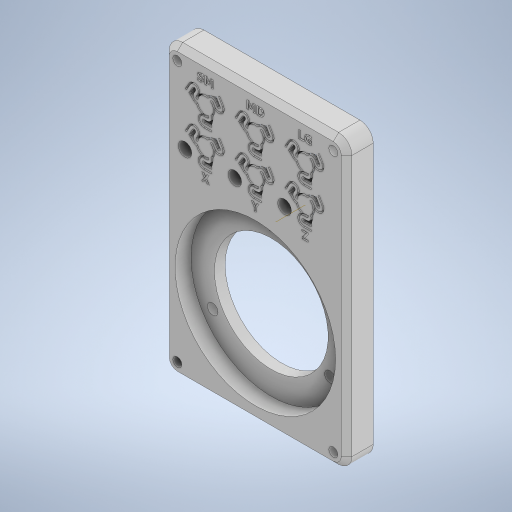
# Autodesk Inventor part: Case Front
Saved by Autodesk Inventor 2023.1 (Build 271208000, 208)
## iProperties
Created: 2022-10-09
Part Number: Case Front
Material: Generic
Document SubType Name: Modeling
Designer: Nick
Density: 1 g/cm^3
Appearance: Default
Author: Nick
Autodesk Inventor part; units mm, degrees
(part 1 of 3)
ref_plane "YZ Plane" through (0, 0, 0) normal (1, 0, 0) x (0, 1, 0)
ref_plane "XZ Plane" through (0, 0, 0) normal (0, 1, 0) x (-1, 0, 0)
ref_plane "XY Plane" through (0, 0, 0) normal (0, 0, 1) x (1, 0, 0)
sketch "Sketch1" plane through (0, 0, 0) normal (0, 0, 1) x (1, 0, 0)
  line L0 (0, 0) -> (68.58, 0)
  line L1 (68.58, 0) -> (68.58, 107.95)
  line L2 (68.58, 107.95) -> (0, 107.95)
  line L3 (0, 107.95) -> (0, 0)
  dimension "d0" = 68.58
  dimension "d1" = 107.95
  constraints: 8 end point, 2 parallel, 1 horizontal, 1 perpendicular
  measures "d0" distance of L2.end L1.end
  measures "d1" distance of L1.end L0.end
extrude "Extrusion1" add sketch "Sketch1" along normal blind 10
sketch "Sketch2" plane through (0, 0, 10) normal (0, 0, 1) x (1, 0, 0)
  circle A0 centre (34.29, 35.56) radius 30.149
  line L0 (0, 0) -> (68.58, 0) projected
  point P0 (34.29, 0)
  dimension "d4" = 60.298
  dimension "d5" = 35.56
  constraints: 1 centre point, 1 midpoint, 1 vertical alignment
  measures "d4" diameter of A0
  measures "d5" distance from line of L0 A0.centre
extrude "Extrusion2" cut sketch "Sketch2" against normal blind 16.9875
sketch "Sketch3" plane through (0, 0, 0) normal (0, 0, -1) x (-1, 0, 0)
  circle A0 centre (-34.29, 35.56) radius 30.149 projected
  circle A1 centre (-34.29, 35.56) radius 21.3606
  point P0 (0, 0)
  dimension "d8" = 42.7212
  constraints: 1 centre point, 1 coincident
  measures "d8" diameter of A1
extrude "Extrusion3" add sketch "Sketch3" against normal blind 4
sketch "Sketch4" plane through (0, 0, 10) normal (0, 0, 1) x (1, 0, 0)
  circle A0 centre (15.59, 80.0195) radius 3
  circle A1 centre (34.29, 80.0195) radius 3
  circle A2 centre (52.99, 93.6395) radius 3
  circle A3 centre (34.29, 93.6395) radius 3
  circle A4 centre (15.59, 93.6395) radius 3
  line L0 (12.59, 96.6395) -> (18.59, 96.6395) construction
  line L1 (18.59, 96.6395) -> (18.59, 90.6395) construction
  line L2 (18.59, 90.6395) -> (12.59, 90.6395) construction
  line L3 (12.59, 90.6395) -> (12.59, 96.6395) construction
  line L4 (31.29, 96.6395) -> (37.29, 96.6395) construction
  line L5 (37.29, 96.6395) -> (37.29, 90.6395) construction
  line L6 (37.29, 90.6395) -> (31.29, 90.6395) construction
  line L7 (31.29, 90.6395) -> (31.29, 96.6395) construction
  line L8 (49.99, 96.6395) -> (55.99, 96.6395) construction
  line L9 (55.99, 96.6395) -> (55.99, 90.6395) construction
  line L10 (55.99, 90.6395) -> (49.99, 90.6395) construction
  line L11 (49.99, 90.6395) -> (49.99, 96.6395) construction
  line L12 (31.29, 83.0195) -> (37.29, 83.0195) construction
  line L13 (37.29, 83.0195) -> (37.29, 77.0195) construction
  line L14 (37.29, 77.0195) -> (31.29, 77.0195) construction
  line L15 (31.29, 77.0195) -> (31.29, 83.0195) construction
  line L16 (12.59, 83.0195) -> (18.59, 83.0195) construction
  line L17 (18.59, 83.0195) -> (18.59, 77.0195) construction
  line L18 (18.59, 77.0195) -> (12.59, 77.0195) construction
  line L19 (12.59, 77.0195) -> (12.59, 83.0195) construction
  line L20 (68.58, 107.95) -> (0, 107.95) construction
  line L21 (17.8543, 65.709) -> (37.2658, 65.709) construction
  circle A5 centre (34.29, 35.56) radius 30.149 construction
  line L22 (27.9805, 81.0411) -> (29.433, 83.5569)
  line L23 (30.7639, 81.3221) -> (31.3989, 82.4219)
  line L24 (27.1145, 81.5411) -> (28.567, 84.0569)
  line L25 (29.8978, 81.8221) -> (30.5328, 82.9219)
  arc A6 (31.3989, 82.4219) -> (28.567, 84.0569) centre (29.9829, 83.2394) ccw
  arc A7 (30.5328, 82.9219) -> (29.433, 83.5569) centre (29.9829, 83.2394) ccw
  arc A8 (29.8978, 81.8221) -> (31.3611, 79.3703) centre (31.3138, 81.0046) ccw
  arc A9 (30.7639, 81.3221) -> (31.3105, 80.3696) centre (31.3138, 81.0046) ccw
  line L26 (34.29, 80.0195) -> (31.0814, 81.872) construction
  line L27 (34.29, 83.0195) -> (34.29, 80.0195) construction
  line L28 (27.1145, 81.5411) -> (27.9805, 81.0411)
  line L29 (26.6814, 81.7911) -> (28.4135, 80.7911)
  line L30 (28.4135, 80.7911) -> (29.866, 83.3069)
  line L31 (30.0998, 83.1719) -> (29.4648, 82.0721)
  arc A10 (30.0998, 83.1719) -> (29.866, 83.3069) centre (29.9829, 83.2394) ccw
  arc A11 (29.4648, 82.0721) -> (31.5152, 78.8791) centre (31.3138, 81.0046) ccw
  arc A12 (31.8319, 82.1719) -> (28.1339, 84.3069) centre (29.9829, 83.2394) ccw
  arc A13 (31.1969, 81.0721) -> (31.442, 80.9622) centre (31.3138, 81.0046) ccw
  line L32 (31.1969, 81.0721) -> (31.8319, 82.1719)
  line L33 (28.1339, 84.3069) -> (26.6814, 81.7911)
  circle A14 centre (52.99, 80.0195) radius 3
  line L34 (49.99, 83.0195) -> (55.99, 83.0195) construction
  line L35 (55.99, 83.0195) -> (55.99, 77.0195) construction
  line L36 (55.99, 77.0195) -> (49.99, 77.0195) construction
  line L37 (49.99, 77.0195) -> (49.99, 83.0195) construction
  line L38 (46.6805, 81.0411) -> (48.133, 83.5569)
  line L39 (49.4639, 81.3221) -> (50.0989, 82.4219)
  line L40 (45.8145, 81.5411) -> (47.267, 84.0569)
  line L41 (48.5978, 81.8221) -> (49.2328, 82.9219)
  arc A15 (50.0989, 82.4219) -> (47.267, 84.0569) centre (48.6829, 83.2394) ccw
  arc A16 (49.2328, 82.9219) -> (48.133, 83.5569) centre (48.6829, 83.2394) ccw
  arc A17 (48.5978, 81.8221) -> (50.0611, 79.3703) centre (50.0138, 81.0046) ccw
  arc A18 (49.4639, 81.3221) -> (50.0105, 80.3696) centre (50.0138, 81.0046) ccw
  line L42 (52.99, 80.0195) -> (49.7814, 81.872) construction
  line L43 (52.99, 83.0195) -> (52.99, 80.0195) construction
  line L44 (45.8145, 81.5411) -> (46.6805, 81.0411)
  line L45 (45.3814, 81.7911) -> (47.1135, 80.7911)
  line L46 (47.1135, 80.7911) -> (48.566, 83.3069)
  line L47 (48.7998, 83.1719) -> (48.1648, 82.0721)
  arc A19 (48.7998, 83.1719) -> (48.566, 83.3069) centre (48.6829, 83.2394) ccw
  arc A20 (48.1648, 82.0721) -> (50.2152, 78.8791) centre (50.0138, 81.0046) ccw
  arc A21 (50.5319, 82.1719) -> (46.8339, 84.3069) centre (48.6829, 83.2394) ccw
  arc A22 (49.8969, 81.0721) -> (50.142, 80.9622) centre (50.0138, 81.0046) ccw
  line L48 (49.8969, 81.0721) -> (50.5319, 82.1719)
  line L49 (46.8339, 84.3069) -> (45.3814, 81.7911)
  circle A23 centre (52.99, 80.0195) radius 3.508
  line L50 (47.1135, 80.7911) -> (48.557, 79.4438)
  point P0 (0, 0)
  point P1 (37.29, 80.0195)
  point P2 (18.59, 80.0195)
  point P3 (18.59, 93.6395)
  point P4 (31.29, 93.6395)
  point P5 (55.99, 93.6395)
  point P6 (34.29, 96.6395)
  point P7 (52.99, 96.6395)
  point P8 (15.59, 96.6395)
  point P9 (15.59, 83.0195)
  point P10 (34.29, 107.95)
  point P11 (27.5475, 81.2911)
  point P12 (55.99, 80.0195)
  point P13 (46.2475, 81.2911)
  point P14 (49.6661, 78.8981)
  point P15 (50.7545, 82.7229)
  point P16 (46.0107, 79.4247)
  dimension "d11" = 7.62
  dimension "d12" = 6
  dimension "d13" = 6
  dimension "d14" = 12.7
  dimension "d15" = 12.7
  dimension "d16" = 11.3105
  dimension "d17" = 11.3105
  dimension "d18" = 1
  dimension "d19" = 60
  dimension "d23" = 1.27
  dimension "d24" = 0.635
  dimension "d25" = 0.5
  dimension "d34" = 6
  dimension "d35" = 6
  dimension "d36" = 1
  dimension "d37" = 60
  dimension "d38" = 1.27
  dimension "d39" = 0.635
  dimension "d40" = 0.5
  dimension "d58" = 0.508
  constraints: 100 end point, 41 point on circle, 30 tangent, 26 parallel, 23 centre point, 19 midpoint, 12 concentric, 10 equal length, 10 perpendicular, 7 collinear, 7 horizontal, 7 vertical alignment, 6 equal radius, 6 horizontal alignment, 2 point on line, 2 vertical
  measures "d11" distance between parallel lines of L12 L6
  measures "d12" distance of L12.start L12.end
  measures "d13" diameter of A1
  measures "d14" distance between parallel lines of L11 L5
  measures "d15" distance between parallel lines of L1 L7
  measures "d16" distance between parallel lines of L20 L4
  measures "d17" distance between parallel lines of L21 L14
  measures "d18" distance between parallel lines of L23 L25
  measures "d19" angle of L27 L26
  measures "d23" distance of L25.start L25.end
  measures "d24" radius of A9
  measures "d25" distance between parallel lines of L30 L22
  measures "d34" distance of L37.end L35.start
  measures "d35" diameter of A14
  measures "d36" distance between parallel lines of L39 L41
  measures "d37" angle of L43 L42
  measures "d38" distance of L41.start L41.end
  measures "d39" radius of A18
  measures "d40" distance between parallel lines of L46 L38
  measures "d58" radial gap between concentric circles of A14 A23
extrude "Extrusion5" cut sketch "Sketch4" against normal through all contours A14 A18 A23 A21 L48 A22 | A20 A23 A17 A14 | A20 L47 A19 L46 L45 L38 A16 L41 A17 A23 | A18 L39 A15 L40 L45 L49 A21 A23 | L50 L46 A19 L47 A20
pattern_circular "Circular Pattern2" count 3 over 360 about axis through (52.99, 80.0195, 10) along (0, 0, 1) of "Extrusion5"
sketch "Sketch6" plane through (0, 0, 10) normal (0, 0, 1) x (1, 0, 0)
  arc A0 (53.8922, 82.8806) -> (53.3898, 82.9927) centre (52.99, 80.0195) ccw projected
  arc A1 (54.7079, 84.1464) -> (53.3898, 82.9927) centre (55.3312, 82.1044) ccw projected
  line L0 (56.5965, 84.7229) -> (57.0295, 84.9729) projected
  line L1 (57.0295, 84.9729) -> (58.482, 82.4571) projected
  arc A2 (57.3822, 81.8221) -> (58.482, 82.4571) centre (57.9321, 82.1396) ccw projected
  line L2 (57.3822, 81.8221) -> (56.7472, 82.9219) projected
  arc A3 (56.7472, 82.9219) -> (53.8922, 82.8806) centre (55.3312, 82.1044) ccw projected
  arc A4 (55.2304, 82.0147) -> (54.7829, 82.4248) centre (52.99, 80.0195) ccw projected
  arc A5 (55.8811, 82.4219) -> (54.7829, 82.4248) centre (55.3312, 82.1044) ccw projected
  line L3 (55.8811, 82.4219) -> (56.5161, 81.3221) projected
  arc A6 (56.5161, 81.3221) -> (59.348, 82.9571) centre (57.9321, 82.1396) ccw projected
  line L4 (59.348, 82.9571) -> (57.8955, 85.4729) projected
  line L5 (57.8955, 85.4729) -> (58.3286, 85.7229) projected
  line L6 (58.3286, 85.7229) -> (59.7811, 83.2071) projected
  arc A7 (56.0831, 81.0721) -> (59.7811, 83.2071) centre (57.9321, 82.1396) ccw projected
  line L7 (56.0831, 81.0721) -> (55.4481, 82.1719) projected
  arc A8 (55.4481, 82.1719) -> (55.2304, 82.0147) centre (55.3312, 82.1044) ccw projected
  arc A9 (55.0167, 77.8076) -> (55.365, 78.1867) centre (52.99, 80.0195) ccw projected
  arc A10 (55.7051, 76.4683) -> (55.365, 78.1867) centre (53.625, 76.9495) ccw projected
  line L8 (55.26, 74.5445) -> (55.26, 74.0445) projected
  line L9 (55.26, 74.0445) -> (52.355, 74.0445) projected
  arc A11 (52.355, 75.3145) -> (52.355, 74.0445) centre (52.355, 74.6795) ccw projected
  line L10 (52.355, 75.3145) -> (53.625, 75.3145) projected
  arc A12 (53.625, 75.3145) -> (55.0167, 77.8076) centre (53.625, 76.9495) ccw projected
  arc A13 (53.5977, 77.0817) -> (54.1766, 77.2641) centre (52.99, 80.0195) ccw projected
  arc A14 (53.625, 76.3145) -> (54.1766, 77.2641) centre (53.625, 76.9495) ccw projected
  line L11 (53.625, 76.3145) -> (52.355, 76.3145) projected
  arc A15 (52.355, 76.3145) -> (52.355, 73.0445) centre (52.355, 74.6795) ccw projected
  line L12 (52.355, 73.0445) -> (55.26, 73.0445) projected
  line L13 (55.26, 73.0445) -> (55.26, 72.5445) projected
  line L14 (55.26, 72.5445) -> (52.355, 72.5445) projected
  arc A16 (52.355, 76.8145) -> (52.355, 72.5445) centre (52.355, 74.6795) ccw projected
  line L15 (52.355, 76.8145) -> (53.625, 76.8145) projected
  arc A17 (53.625, 76.8145) -> (53.5977, 77.0817) centre (53.625, 76.9495) ccw projected
  line L16 (47.1135, 80.7911) -> (46.6805, 81.0411) projected
  line L17 (46.6805, 81.0411) -> (48.133, 83.5569) projected
  arc A18 (49.2328, 82.9219) -> (48.133, 83.5569) centre (48.6829, 83.2394) ccw projected
  line L18 (49.2328, 82.9219) -> (48.5978, 81.8221) projected
  arc A19 (48.5978, 81.8221) -> (50.0611, 79.3703) centre (50.0138, 81.0046) ccw projected
  arc A20 (50.0611, 79.3703) -> (50.2152, 78.8791) centre (52.99, 80.0195) ccw projected
  arc A21 (48.557, 79.4438) -> (50.2152, 78.8791) centre (50.0138, 81.0046) ccw projected
  line L19 (47.267, 84.0569) -> (45.8145, 81.5411) projected
  line L20 (45.8145, 81.5411) -> (45.3814, 81.7911) projected
  line L21 (45.3814, 81.7911) -> (46.8339, 84.3069) projected
  arc A22 (50.5319, 82.1719) -> (46.8339, 84.3069) centre (48.6829, 83.2394) ccw projected
  line L22 (50.5319, 82.1719) -> (49.8969, 81.0721) projected
  arc A23 (49.8969, 81.0721) -> (50.142, 80.9622) centre (50.0138, 81.0046) ccw projected
  arc A24 (50.142, 80.9622) -> (50.0105, 80.3696) centre (52.99, 80.0195) ccw projected
  arc A25 (49.4639, 81.3221) -> (50.0105, 80.3696) centre (50.0138, 81.0046) ccw projected
  line L23 (49.4639, 81.3221) -> (50.0989, 82.4219) projected
  arc A26 (50.0989, 82.4219) -> (47.267, 84.0569) centre (48.6829, 83.2394) ccw projected
  circle A27 centre (34.29, 35.56) radius 30.149 projected
  line L24 (68.58, 0) -> (68.58, 107.95) projected
  line L25 (68.58, 107.95) -> (0, 107.95) projected
  line L26 (0, 107.95) -> (0, 0) projected
  line L27 (0, 0) -> (68.58, 0) projected
  circle A28 centre (52.99, 80.0195) radius 3
  circle A29 centre (52.99, 80.0195) radius 3.508
  line L28 (54.7079, 84.1464) -> (56.5965, 84.7229) projected
  line L29 (55.7051, 76.4683) -> (55.26, 74.5445) projected
  line L30 (48.557, 79.4438) -> (47.1135, 80.7911) projected
  point P0 (53.5977, 77.0817)
  point P1 (50.2152, 78.8791)
  point P2 (49.6661, 78.8981)
  point P3 (51.7665, 76.7318)
  point P4 (55.2304, 82.0147)
  point P5 (55.365, 78.1867)
  point P6 (55.6231, 77.7016)
  point P7 (56.449, 80.6038)
  point P8 (50.142, 80.9622)
  point P9 (53.3898, 82.9927)
  point P10 (53.6808, 83.4588)
  point P11 (50.7545, 82.7229)
  dimension "d59" = 6
  dimension "d60" = 0.508
  constraints: 2 centre point, 1 coincident
  measures "d59" diameter of A28
  measures "d60" radial gap between concentric circles of A28 A29
extrude "Extrusion7" cut sketch "Sketch6" against normal through all contours A28 A23 L22 A22 A29 A1 | A8 L7 A7 A29 A10 A28 | A28 A17 L15 A16 A29 A21
pattern_linear "Rectangular Pattern2" count 3 spacing 18.7 along (-1, 0, 0) count 2 spacing 13.62 along (0, 1, 0) of "Extrusion5", "Circular Pattern2", "Extrusion7"
sketch "Sketch5" plane through (0, 0, 0) normal (0, 0, -1) x (-1, 0, 0)
  line L0 (-66.58, 105.95) -> (-2, 105.95)
  line L1 (-2, 105.95) -> (-2, 65.9374)
  line L2 (-2, 65.9374) -> (-66.58, 65.9374)
  line L3 (-66.58, 65.9374) -> (-66.58, 105.95)
  line L4 (-68.58, 107.95) -> (0, 107.95) projected
  line L5 (0, 107.95) -> (0, 0) projected
  line L6 (-68.58, 0) -> (-68.58, 107.95) projected
  line L7 (-14.955, 72.5445) -> (-17.86, 72.5445) projected
  point P0 (-20.9286, 99.3429)
  dimension "d52" = 2
  dimension "d53" = 2
  dimension "d54" = 2
  dimension "d74" = 6.6071
  dimension "d75" = 6.6071
  constraints: 8 end point, 2 parallel, 1 horizontal, 1 perpendicular
  measures "d52" distance between parallel lines of L4 L0
  measures "d53" distance between parallel lines of L5 L1
  measures "d54" distance between parallel lines of L6 L3
  measures "d74" distance from line of L0 point (-20.929, 99.343)
  measures "d75" distance between parallel lines of L2 L7
extrude "Extrusion6" cut sketch "Sketch5" against normal blind 9
sketch "Sketch7" plane through (0, 0, 10) normal (0, 0, 1) x (1, 0, 0)
  line L0 (11.8335, 71.5445) -> (19.3465, 71.5445) construction
  line L1 (19.3465, 71.5445) -> (19.3465, 68.4965) construction
  line L2 (19.3465, 68.4965) -> (11.8335, 68.4965) construction
  line L3 (11.8335, 68.4965) -> (11.8335, 71.5445) construction
  line L4 (30.5175, 71.5445) -> (38.0625, 71.5445) construction
  line L5 (38.0625, 71.5445) -> (38.0625, 68.4965) construction
  line L6 (38.0625, 68.4965) -> (30.5175, 68.4965) construction
  line L7 (30.5175, 68.4965) -> (30.5175, 71.5445) construction
  line L8 (54.358, 71.5445) -> (51.622, 71.5445) construction
  line L9 (51.622, 71.5445) -> (51.622, 68.4965) construction
  line L10 (51.622, 68.4965) -> (54.358, 68.4965) construction
  line L11 (54.358, 68.4965) -> (54.358, 71.5445) construction
  line L12 (12.8075, 103.4996) -> (18.3725, 103.4996) construction
  line L13 (18.3725, 103.4996) -> (18.3725, 100.3429) construction
  line L14 (18.3725, 100.3429) -> (12.8075, 100.3429) construction
  line L15 (12.8075, 100.3429) -> (12.8075, 103.4996) construction
  line L16 (31.2531, 103.3909) -> (37.3269, 103.3909) construction
  line L17 (37.3269, 103.3909) -> (37.3269, 100.3429) construction
  line L18 (37.3269, 100.3429) -> (31.2531, 100.3429) construction
  line L19 (31.2531, 100.3429) -> (31.2531, 103.3909) construction
  line L20 (50.5484, 103.5045) -> (55.4316, 103.5045) construction
  line L21 (55.4316, 103.5045) -> (55.4316, 100.3429) construction
  line L22 (55.4316, 100.3429) -> (50.5484, 100.3429) construction
  line L23 (50.5484, 100.3429) -> (50.5484, 103.5045) construction
  line L24 (68.58, 0) -> (68.58, 107.95) projected
  line L25 (68.58, 107.95) -> (0, 107.95) projected
  line L26 (0, 107.95) -> (0, 0) projected
  line L27 (0, 0) -> (68.58, 0) projected
  circle A0 centre (34.29, 35.56) radius 30.149 projected
  arc A1 (53.6808, 83.4588) -> (50.7545, 82.7229) centre (52.99, 80.0195) ccw projected
  arc A2 (54.7079, 84.1464) -> (53.6808, 83.4588) centre (55.3312, 82.1044) ccw projected
  line L28 (56.5965, 84.7229) -> (57.0295, 84.9729) projected
  line L29 (57.0295, 84.9729) -> (58.482, 82.4571) projected
  arc A3 (57.3822, 81.8221) -> (58.482, 82.4571) centre (57.9321, 82.1396) ccw projected
  line L30 (57.3822, 81.8221) -> (56.7472, 82.9219) projected
  arc A4 (56.7472, 82.9219) -> (53.8922, 82.8806) centre (55.3312, 82.1044) ccw projected
  arc A5 (53.8922, 82.8806) -> (50.0105, 80.3696) centre (52.99, 80.0195) ccw projected
  arc A6 (49.4639, 81.3221) -> (50.0105, 80.3696) centre (50.0138, 81.0046) ccw projected
  line L31 (49.4639, 81.3221) -> (50.0989, 82.4219) projected
  arc A7 (50.0989, 82.4219) -> (47.267, 84.0569) centre (48.6829, 83.2394) ccw projected
  line L32 (47.267, 84.0569) -> (45.8145, 81.5411) projected
  line L33 (45.8145, 81.5411) -> (45.3814, 81.7911) projected
  line L34 (45.3814, 81.7911) -> (46.8339, 84.3069) projected
  arc A8 (50.7545, 82.7229) -> (46.8339, 84.3069) centre (48.6829, 83.2394) ccw projected
  arc A9 (55.6231, 77.7016) -> (56.449, 80.6038) centre (52.99, 80.0195) ccw projected
  arc A10 (55.7051, 76.4683) -> (55.6231, 77.7016) centre (53.625, 76.9495) ccw projected
  line L35 (55.26, 74.5445) -> (55.26, 74.0445) projected
  line L36 (55.26, 74.0445) -> (52.355, 74.0445) projected
  arc A11 (52.355, 75.3145) -> (52.355, 74.0445) centre (52.355, 74.6795) ccw projected
  line L37 (52.355, 75.3145) -> (53.625, 75.3145) projected
  arc A12 (53.625, 75.3145) -> (55.0167, 77.8076) centre (53.625, 76.9495) ccw projected
  arc A13 (55.0167, 77.8076) -> (54.7829, 82.4248) centre (52.99, 80.0195) ccw projected
  arc A14 (55.8811, 82.4219) -> (54.7829, 82.4248) centre (55.3312, 82.1044) ccw projected
  line L38 (55.8811, 82.4219) -> (56.5161, 81.3221) projected
  arc A15 (56.5161, 81.3221) -> (59.348, 82.9571) centre (57.9321, 82.1396) ccw projected
  line L39 (59.348, 82.9571) -> (57.8955, 85.4729) projected
  line L40 (57.8955, 85.4729) -> (58.3286, 85.7229) projected
  line L41 (58.3286, 85.7229) -> (59.7811, 83.2071) projected
  arc A16 (56.449, 80.6038) -> (59.7811, 83.2071) centre (57.9321, 82.1396) ccw projected
  arc A17 (49.6661, 78.8981) -> (51.7665, 76.7318) centre (52.99, 80.0195) ccw projected
  arc A18 (48.557, 79.4438) -> (49.6661, 78.8981) centre (50.0138, 81.0046) ccw projected
  line L42 (47.1135, 80.7911) -> (46.6805, 81.0411) projected
  line L43 (46.6805, 81.0411) -> (48.133, 83.5569) projected
  arc A19 (49.2328, 82.9219) -> (48.133, 83.5569) centre (48.6829, 83.2394) ccw projected
  line L44 (49.2328, 82.9219) -> (48.5978, 81.8221) projected
  arc A20 (48.5978, 81.8221) -> (50.0611, 79.3703) centre (50.0138, 81.0046) ccw projected
  arc A21 (50.0611, 79.3703) -> (54.1766, 77.2641) centre (52.99, 80.0195) ccw projected
  arc A22 (53.625, 76.3145) -> (54.1766, 77.2641) centre (53.625, 76.9495) ccw projected
  line L45 (53.625, 76.3145) -> (52.355, 76.3145) projected
  arc A23 (52.355, 76.3145) -> (52.355, 73.0445) centre (52.355, 74.6795) ccw projected
  line L46 (52.355, 73.0445) -> (55.26, 73.0445) projected
  line L47 (55.26, 73.0445) -> (55.26, 72.5445) projected
  line L48 (55.26, 72.5445) -> (52.355, 72.5445) projected
  arc A24 (51.7665, 76.7318) -> (52.355, 72.5445) centre (52.355, 74.6795) ccw projected
  arc A25 (31.3611, 79.3703) -> (35.4766, 77.2641) centre (34.29, 80.0195) ccw projected
  arc A26 (34.925, 76.3145) -> (35.4766, 77.2641) centre (34.925, 76.9495) ccw projected
  line L49 (34.925, 76.3145) -> (33.655, 76.3145) projected
  arc A27 (33.655, 76.3145) -> (33.655, 73.0445) centre (33.655, 74.6795) ccw projected
  line L50 (33.655, 73.0445) -> (36.56, 73.0445) projected
  line L51 (36.56, 73.0445) -> (36.56, 72.5445) projected
  line L52 (36.56, 72.5445) -> (33.655, 72.5445) projected
  arc A28 (33.0665, 76.7318) -> (33.655, 72.5445) centre (33.655, 74.6795) ccw projected
  arc A29 (30.9661, 78.8981) -> (33.0665, 76.7318) centre (34.29, 80.0195) ccw projected
  arc A30 (29.857, 79.4438) -> (30.9661, 78.8981) centre (31.3138, 81.0046) ccw projected
  line L53 (28.4135, 80.7911) -> (27.9805, 81.0411) projected
  line L54 (27.9805, 81.0411) -> (29.433, 83.5569) projected
  arc A31 (30.5328, 82.9219) -> (29.433, 83.5569) centre (29.9829, 83.2394) ccw projected
  line L55 (30.5328, 82.9219) -> (29.8978, 81.8221) projected
  arc A32 (29.8978, 81.8221) -> (31.3611, 79.3703) centre (31.3138, 81.0046) ccw projected
  arc A33 (36.3167, 77.8076) -> (36.0829, 82.4248) centre (34.29, 80.0195) ccw projected
  arc A34 (37.1811, 82.4219) -> (36.0829, 82.4248) centre (36.6312, 82.1044) ccw projected
  line L56 (37.1811, 82.4219) -> (37.8161, 81.3221) projected
  arc A35 (37.8161, 81.3221) -> (40.648, 82.9571) centre (39.2321, 82.1396) ccw projected
  line L57 (40.648, 82.9571) -> (39.1955, 85.4729) projected
  line L58 (39.1955, 85.4729) -> (39.6286, 85.7229) projected
  line L59 (39.6286, 85.7229) -> (41.0811, 83.2071) projected
  arc A36 (37.749, 80.6038) -> (41.0811, 83.2071) centre (39.2321, 82.1396) ccw projected
  arc A37 (36.9231, 77.7016) -> (37.749, 80.6038) centre (34.29, 80.0195) ccw projected
  arc A38 (37.0051, 76.4683) -> (36.9231, 77.7016) centre (34.925, 76.9495) ccw projected
  line L60 (36.56, 74.5445) -> (36.56, 74.0445) projected
  line L61 (36.56, 74.0445) -> (33.655, 74.0445) projected
  arc A39 (33.655, 75.3145) -> (33.655, 74.0445) centre (33.655, 74.6795) ccw projected
  line L62 (33.655, 75.3145) -> (34.925, 75.3145) projected
  arc A40 (34.925, 75.3145) -> (36.3167, 77.8076) centre (34.925, 76.9495) ccw projected
  arc A41 (34.9808, 83.4588) -> (32.0545, 82.7229) centre (34.29, 80.0195) ccw projected
  arc A42 (36.0079, 84.1464) -> (34.9808, 83.4588) centre (36.6312, 82.1044) ccw projected
  line L63 (37.8965, 84.7229) -> (38.3295, 84.9729) projected
  line L64 (38.3295, 84.9729) -> (39.782, 82.4571) projected
  arc A43 (38.6822, 81.8221) -> (39.782, 82.4571) centre (39.2321, 82.1396) ccw projected
  line L65 (38.6822, 81.8221) -> (38.0472, 82.9219) projected
  arc A44 (38.0472, 82.9219) -> (35.1922, 82.8806) centre (36.6312, 82.1044) ccw projected
  arc A45 (35.1922, 82.8806) -> (31.3105, 80.3696) centre (34.29, 80.0195) ccw projected
  arc A46 (30.7639, 81.3221) -> (31.3105, 80.3696) centre (31.3138, 81.0046) ccw projected
  line L66 (30.7639, 81.3221) -> (31.3989, 82.4219) projected
  arc A47 (31.3989, 82.4219) -> (28.567, 84.0569) centre (29.9829, 83.2394) ccw projected
  line L67 (28.567, 84.0569) -> (27.1145, 81.5411) projected
  line L68 (27.1145, 81.5411) -> (26.6814, 81.7911) projected
  line L69 (26.6814, 81.7911) -> (28.1339, 84.3069) projected
  arc A48 (32.0545, 82.7229) -> (28.1339, 84.3069) centre (29.9829, 83.2394) ccw projected
  arc A49 (12.6611, 79.3703) -> (16.7766, 77.2641) centre (15.59, 80.0195) ccw projected
  arc A50 (16.225, 76.3145) -> (16.7766, 77.2641) centre (16.225, 76.9495) ccw projected
  line L70 (16.225, 76.3145) -> (14.955, 76.3145) projected
  arc A51 (14.955, 76.3145) -> (14.955, 73.0445) centre (14.955, 74.6795) ccw projected
  line L71 (14.955, 73.0445) -> (17.86, 73.0445) projected
  line L72 (17.86, 73.0445) -> (17.86, 72.5445) projected
  line L73 (17.86, 72.5445) -> (14.955, 72.5445) projected
  arc A52 (14.3665, 76.7318) -> (14.955, 72.5445) centre (14.955, 74.6795) ccw projected
  arc A53 (12.2661, 78.8981) -> (14.3665, 76.7318) centre (15.59, 80.0195) ccw projected
  arc A54 (11.157, 79.4438) -> (12.2661, 78.8981) centre (12.6138, 81.0046) ccw projected
  line L74 (9.7135, 80.7911) -> (9.2805, 81.0411) projected
  line L75 (9.2805, 81.0411) -> (10.733, 83.5569) projected
  arc A55 (11.8328, 82.9219) -> (10.733, 83.5569) centre (11.2829, 83.2394) ccw projected
  line L76 (11.8328, 82.9219) -> (11.1978, 81.8221) projected
  arc A56 (11.1978, 81.8221) -> (12.6611, 79.3703) centre (12.6138, 81.0046) ccw projected
  arc A57 (17.6167, 77.8076) -> (17.3829, 82.4248) centre (15.59, 80.0195) ccw projected
  arc A58 (18.4811, 82.4219) -> (17.3829, 82.4248) centre (17.9312, 82.1044) ccw projected
  line L77 (18.4811, 82.4219) -> (19.1161, 81.3221) projected
  arc A59 (19.1161, 81.3221) -> (21.948, 82.9571) centre (20.5321, 82.1396) ccw projected
  line L78 (21.948, 82.9571) -> (20.4955, 85.4729) projected
  line L79 (20.4955, 85.4729) -> (20.9286, 85.7229) projected
  line L80 (20.9286, 85.7229) -> (22.3811, 83.2071) projected
  arc A60 (19.049, 80.6038) -> (22.3811, 83.2071) centre (20.5321, 82.1396) ccw projected
  arc A61 (18.2231, 77.7016) -> (19.049, 80.6038) centre (15.59, 80.0195) ccw projected
  arc A62 (18.3051, 76.4683) -> (18.2231, 77.7016) centre (16.225, 76.9495) ccw projected
  line L81 (17.86, 74.5445) -> (17.86, 74.0445) projected
  line L82 (17.86, 74.0445) -> (14.955, 74.0445) projected
  arc A63 (14.955, 75.3145) -> (14.955, 74.0445) centre (14.955, 74.6795) ccw projected
  line L83 (14.955, 75.3145) -> (16.225, 75.3145) projected
  arc A64 (16.225, 75.3145) -> (17.6167, 77.8076) centre (16.225, 76.9495) ccw projected
  arc A65 (16.2808, 83.4588) -> (13.3545, 82.7229) centre (15.59, 80.0195) ccw projected
  arc A66 (17.3079, 84.1464) -> (16.2808, 83.4588) centre (17.9312, 82.1044) ccw projected
  line L84 (19.1965, 84.7229) -> (19.6295, 84.9729) projected
  line L85 (19.6295, 84.9729) -> (21.082, 82.4571) projected
  arc A67 (19.9822, 81.8221) -> (21.082, 82.4571) centre (20.5321, 82.1396) ccw projected
  line L86 (19.9822, 81.8221) -> (19.3472, 82.9219) projected
  arc A68 (19.3472, 82.9219) -> (16.4922, 82.8806) centre (17.9312, 82.1044) ccw projected
  arc A69 (16.4922, 82.8806) -> (12.6105, 80.3696) centre (15.59, 80.0195) ccw projected
  arc A70 (12.0639, 81.3221) -> (12.6105, 80.3696) centre (12.6138, 81.0046) ccw projected
  line L87 (12.0639, 81.3221) -> (12.6989, 82.4219) projected
  arc A71 (12.6989, 82.4219) -> (9.867, 84.0569) centre (11.2829, 83.2394) ccw projected
  line L88 (9.867, 84.0569) -> (8.4145, 81.5411) projected
  line L89 (8.4145, 81.5411) -> (7.9814, 81.7911) projected
  line L90 (7.9814, 81.7911) -> (9.4339, 84.3069) projected
  arc A72 (13.3545, 82.7229) -> (9.4339, 84.3069) centre (11.2829, 83.2394) ccw projected
  arc A73 (50.0611, 92.9903) -> (54.1766, 90.8841) centre (52.99, 93.6395) ccw projected
  arc A74 (53.625, 89.9345) -> (54.1766, 90.8841) centre (53.625, 90.5695) ccw projected
  line L91 (53.625, 89.9345) -> (52.355, 89.9345) projected
  arc A75 (52.355, 89.9345) -> (52.355, 86.6645) centre (52.355, 88.2995) ccw projected
  line L92 (52.355, 86.6645) -> (55.26, 86.6645) projected
  line L93 (55.26, 86.6645) -> (55.26, 86.1645) projected
  line L94 (55.26, 86.1645) -> (52.355, 86.1645) projected
  arc A76 (51.7665, 90.3518) -> (52.355, 86.1645) centre (52.355, 88.2995) ccw projected
  arc A77 (49.6661, 92.5181) -> (51.7665, 90.3518) centre (52.99, 93.6395) ccw projected
  arc A78 (48.557, 93.0638) -> (49.6661, 92.5181) centre (50.0138, 94.6246) ccw projected
  line L95 (47.1135, 94.4111) -> (46.6805, 94.6611) projected
  line L96 (46.6805, 94.6611) -> (48.133, 97.1769) projected
  arc A79 (49.2328, 96.5419) -> (48.133, 97.1769) centre (48.6829, 96.8594) ccw projected
  line L97 (49.2328, 96.5419) -> (48.5978, 95.4421) projected
  arc A80 (48.5978, 95.4421) -> (50.0611, 92.9903) centre (50.0138, 94.6246) ccw projected
  arc A81 (55.0167, 91.4276) -> (54.7829, 96.0448) centre (52.99, 93.6395) ccw projected
  arc A82 (55.8811, 96.0419) -> (54.7829, 96.0448) centre (55.3312, 95.7244) ccw projected
  line L98 (55.8811, 96.0419) -> (56.5161, 94.9421) projected
  arc A83 (56.5161, 94.9421) -> (59.348, 96.5771) centre (57.9321, 95.7596) ccw projected
  line L99 (59.348, 96.5771) -> (57.8955, 99.0929) projected
  line L100 (57.8955, 99.0929) -> (58.3286, 99.3429) projected
  line L101 (58.3286, 99.3429) -> (59.7811, 96.8271) projected
  arc A84 (56.449, 94.2238) -> (59.7811, 96.8271) centre (57.9321, 95.7596) ccw projected
  arc A85 (55.6231, 91.3216) -> (56.449, 94.2238) centre (52.99, 93.6395) ccw projected
  arc A86 (55.7051, 90.0883) -> (55.6231, 91.3216) centre (53.625, 90.5695) ccw projected
  line L102 (55.26, 88.1645) -> (55.26, 87.6645) projected
  line L103 (55.26, 87.6645) -> (52.355, 87.6645) projected
  arc A87 (52.355, 88.9345) -> (52.355, 87.6645) centre (52.355, 88.2995) ccw projected
  line L104 (52.355, 88.9345) -> (53.625, 88.9345) projected
  arc A88 (53.625, 88.9345) -> (55.0167, 91.4276) centre (53.625, 90.5695) ccw projected
  arc A89 (53.6808, 97.0788) -> (50.7545, 96.3429) centre (52.99, 93.6395) ccw projected
  arc A90 (54.7079, 97.7664) -> (53.6808, 97.0788) centre (55.3312, 95.7244) ccw projected
  line L105 (56.5965, 98.3429) -> (57.0295, 98.5929) projected
  line L106 (57.0295, 98.5929) -> (58.482, 96.0771) projected
  arc A91 (57.3822, 95.4421) -> (58.482, 96.0771) centre (57.9321, 95.7596) ccw projected
  line L107 (57.3822, 95.4421) -> (56.7472, 96.5419) projected
  arc A92 (56.7472, 96.5419) -> (53.8922, 96.5006) centre (55.3312, 95.7244) ccw projected
  arc A93 (53.8922, 96.5006) -> (50.0105, 93.9896) centre (52.99, 93.6395) ccw projected
  arc A94 (49.4639, 94.9421) -> (50.0105, 93.9896) centre (50.0138, 94.6246) ccw projected
  line L108 (49.4639, 94.9421) -> (50.0989, 96.0419) projected
  arc A95 (50.0989, 96.0419) -> (47.267, 97.6769) centre (48.6829, 96.8594) ccw projected
  line L109 (47.267, 97.6769) -> (45.8145, 95.1611) projected
  line L110 (45.8145, 95.1611) -> (45.3814, 95.4111) projected
  line L111 (45.3814, 95.4111) -> (46.8339, 97.9269) projected
  arc A96 (50.7545, 96.3429) -> (46.8339, 97.9269) centre (48.6829, 96.8594) ccw projected
  arc A97 (31.3611, 92.9903) -> (35.4766, 90.8841) centre (34.29, 93.6395) ccw projected
  arc A98 (34.925, 89.9345) -> (35.4766, 90.8841) centre (34.925, 90.5695) ccw projected
  line L112 (34.925, 89.9345) -> (33.655, 89.9345) projected
  arc A99 (33.655, 89.9345) -> (33.655, 86.6645) centre (33.655, 88.2995) ccw projected
  line L113 (33.655, 86.6645) -> (36.56, 86.6645) projected
  line L114 (36.56, 86.6645) -> (36.56, 86.1645) projected
  line L115 (36.56, 86.1645) -> (33.655, 86.1645) projected
  arc A100 (33.0665, 90.3518) -> (33.655, 86.1645) centre (33.655, 88.2995) ccw projected
  arc A101 (30.9661, 92.5181) -> (33.0665, 90.3518) centre (34.29, 93.6395) ccw projected
  arc A102 (29.857, 93.0638) -> (30.9661, 92.5181) centre (31.3138, 94.6246) ccw projected
  line L116 (28.4135, 94.4111) -> (27.9805, 94.6611) projected
  line L117 (27.9805, 94.6611) -> (29.433, 97.1769) projected
  arc A103 (30.5328, 96.5419) -> (29.433, 97.1769) centre (29.9829, 96.8594) ccw projected
  line L118 (30.5328, 96.5419) -> (29.8978, 95.4421) projected
  arc A104 (29.8978, 95.4421) -> (31.3611, 92.9903) centre (31.3138, 94.6246) ccw projected
  arc A105 (36.3167, 91.4276) -> (36.0829, 96.0448) centre (34.29, 93.6395) ccw projected
  arc A106 (37.1811, 96.0419) -> (36.0829, 96.0448) centre (36.6312, 95.7244) ccw projected
  line L119 (37.1811, 96.0419) -> (37.8161, 94.9421) projected
  arc A107 (37.8161, 94.9421) -> (40.648, 96.5771) centre (39.2321, 95.7596) ccw projected
  line L120 (40.648, 96.5771) -> (39.1955, 99.0929) projected
  line L121 (39.1955, 99.0929) -> (39.6286, 99.3429) projected
  line L122 (39.6286, 99.3429) -> (41.0811, 96.8271) projected
  arc A108 (37.749, 94.2238) -> (41.0811, 96.8271) centre (39.2321, 95.7596) ccw projected
  arc A109 (36.9231, 91.3216) -> (37.749, 94.2238) centre (34.29, 93.6395) ccw projected
  arc A110 (37.0051, 90.0883) -> (36.9231, 91.3216) centre (34.925, 90.5695) ccw projected
  line L123 (36.56, 88.1645) -> (36.56, 87.6645) projected
  line L124 (36.56, 87.6645) -> (33.655, 87.6645) projected
  arc A111 (33.655, 88.9345) -> (33.655, 87.6645) centre (33.655, 88.2995) ccw projected
  line L125 (33.655, 88.9345) -> (34.925, 88.9345) projected
  arc A112 (34.925, 88.9345) -> (36.3167, 91.4276) centre (34.925, 90.5695) ccw projected
  arc A113 (34.9808, 97.0788) -> (32.0545, 96.3429) centre (34.29, 93.6395) ccw projected
  arc A114 (36.0079, 97.7664) -> (34.9808, 97.0788) centre (36.6312, 95.7244) ccw projected
  line L126 (37.8965, 98.3429) -> (38.3295, 98.5929) projected
  line L127 (38.3295, 98.5929) -> (39.782, 96.0771) projected
  arc A115 (38.6822, 95.4421) -> (39.782, 96.0771) centre (39.2321, 95.7596) ccw projected
  line L128 (38.6822, 95.4421) -> (38.0472, 96.5419) projected
  arc A116 (38.0472, 96.5419) -> (35.1922, 96.5006) centre (36.6312, 95.7244) ccw projected
  arc A117 (35.1922, 96.5006) -> (31.3105, 93.9896) centre (34.29, 93.6395) ccw projected
  arc A118 (30.7639, 94.9421) -> (31.3105, 93.9896) centre (31.3138, 94.6246) ccw projected
  line L129 (30.7639, 94.9421) -> (31.3989, 96.0419) projected
  arc A119 (31.3989, 96.0419) -> (28.567, 97.6769) centre (29.9829, 96.8594) ccw projected
  line L130 (28.567, 97.6769) -> (27.1145, 95.1611) projected
  line L131 (27.1145, 95.1611) -> (26.6814, 95.4111) projected
  line L132 (26.6814, 95.4111) -> (28.1339, 97.9269) projected
  arc A120 (32.0545, 96.3429) -> (28.1339, 97.9269) centre (29.9829, 96.8594) ccw projected
  arc A121 (12.6611, 92.9903) -> (16.7766, 90.8841) centre (15.59, 93.6395) ccw projected
  arc A122 (16.225, 89.9345) -> (16.7766, 90.8841) centre (16.225, 90.5695) ccw projected
  line L133 (16.225, 89.9345) -> (14.955, 89.9345) projected
  arc A123 (14.955, 89.9345) -> (14.955, 86.6645) centre (14.955, 88.2995) ccw projected
  line L134 (14.955, 86.6645) -> (17.86, 86.6645) projected
  line L135 (17.86, 86.6645) -> (17.86, 86.1645) projected
  line L136 (17.86, 86.1645) -> (14.955, 86.1645) projected
  arc A124 (14.3665, 90.3518) -> (14.955, 86.1645) centre (14.955, 88.2995) ccw projected
  arc A125 (12.2661, 92.5181) -> (14.3665, 90.3518) centre (15.59, 93.6395) ccw projected
  arc A126 (11.157, 93.0638) -> (12.2661, 92.5181) centre (12.6138, 94.6246) ccw projected
  line L137 (9.7135, 94.4111) -> (9.2805, 94.6611) projected
  line L138 (9.2805, 94.6611) -> (10.733, 97.1769) projected
  arc A127 (11.8328, 96.5419) -> (10.733, 97.1769) centre (11.2829, 96.8594) ccw projected
  line L139 (11.8328, 96.5419) -> (11.1978, 95.4421) projected
  arc A128 (11.1978, 95.4421) -> (12.6611, 92.9903) centre (12.6138, 94.6246) ccw projected
  arc A129 (17.6167, 91.4276) -> (17.3829, 96.0448) centre (15.59, 93.6395) ccw projected
  arc A130 (18.4811, 96.0419) -> (17.3829, 96.0448) centre (17.9312, 95.7244) ccw projected
  line L140 (18.4811, 96.0419) -> (19.1161, 94.9421) projected
  arc A131 (19.1161, 94.9421) -> (21.948, 96.5771) centre (20.5321, 95.7596) ccw projected
  line L141 (21.948, 96.5771) -> (20.4955, 99.0929) projected
  line L142 (20.4955, 99.0929) -> (20.9286, 99.3429) projected
  line L143 (20.9286, 99.3429) -> (22.3811, 96.8271) projected
  arc A132 (19.049, 94.2238) -> (22.3811, 96.8271) centre (20.5321, 95.7596) ccw projected
  arc A133 (18.2231, 91.3216) -> (19.049, 94.2238) centre (15.59, 93.6395) ccw projected
  arc A134 (18.3051, 90.0883) -> (18.2231, 91.3216) centre (16.225, 90.5695) ccw projected
  line L144 (17.86, 88.1645) -> (17.86, 87.6645) projected
  line L145 (17.86, 87.6645) -> (14.955, 87.6645) projected
  arc A135 (14.955, 88.9345) -> (14.955, 87.6645) centre (14.955, 88.2995) ccw projected
  line L146 (14.955, 88.9345) -> (16.225, 88.9345) projected
  arc A136 (16.225, 88.9345) -> (17.6167, 91.4276) centre (16.225, 90.5695) ccw projected
  arc A137 (16.2808, 97.0788) -> (13.3545, 96.3429) centre (15.59, 93.6395) ccw projected
  arc A138 (17.3079, 97.7664) -> (16.2808, 97.0788) centre (17.9312, 95.7244) ccw projected
  line L147 (19.1965, 98.3429) -> (19.6295, 98.5929) projected
  line L148 (19.6295, 98.5929) -> (21.082, 96.0771) projected
  arc A139 (19.9822, 95.4421) -> (21.082, 96.0771) centre (20.5321, 95.7596) ccw projected
  line L149 (19.9822, 95.4421) -> (19.3472, 96.5419) projected
  arc A140 (19.3472, 96.5419) -> (16.4922, 96.5006) centre (17.9312, 95.7244) ccw projected
  arc A141 (16.4922, 96.5006) -> (12.6105, 93.9896) centre (15.59, 93.6395) ccw projected
  arc A142 (12.0639, 94.9421) -> (12.6105, 93.9896) centre (12.6138, 94.6246) ccw projected
  line L150 (12.0639, 94.9421) -> (12.6989, 96.0419) projected
  arc A143 (12.6989, 96.0419) -> (9.867, 97.6769) centre (11.2829, 96.8594) ccw projected
  line L151 (9.867, 97.6769) -> (8.4145, 95.1611) projected
  line L152 (8.4145, 95.1611) -> (7.9814, 95.4111) projected
  line L153 (7.9814, 95.4111) -> (9.4339, 97.9269) projected
  arc A144 (13.3545, 96.3429) -> (9.4339, 97.9269) centre (11.2829, 96.8594) ccw projected
  line L154 (54.7079, 84.1464) -> (56.5965, 84.7229) projected
  line L155 (55.7051, 76.4683) -> (55.26, 74.5445) projected
  line L156 (48.557, 79.4438) -> (47.1135, 80.7911) projected
  line L157 (29.857, 79.4438) -> (28.4135, 80.7911) projected
  line L158 (36.0079, 84.1464) -> (37.8965, 84.7229) projected
  line L159 (37.0051, 76.4683) -> (36.56, 74.5445) projected
  line L160 (11.157, 79.4438) -> (9.7135, 80.7911) projected
  line L161 (17.3079, 84.1464) -> (19.1965, 84.7229) projected
  line L162 (18.3051, 76.4683) -> (17.86, 74.5445) projected
  line L163 (48.557, 93.0638) -> (47.1135, 94.4111) projected
  line L164 (54.7079, 97.7664) -> (56.5965, 98.3429) projected
  line L165 (55.7051, 90.0883) -> (55.26, 88.1645) projected
  line L166 (29.857, 93.0638) -> (28.4135, 94.4111) projected
  line L167 (36.0079, 97.7664) -> (37.8965, 98.3429) projected
  line L168 (37.0051, 90.0883) -> (36.56, 88.1645) projected
  line L169 (11.157, 93.0638) -> (9.7135, 94.4111) projected
  line L170 (17.3079, 97.7664) -> (19.1965, 98.3429) projected
  line L171 (18.3051, 90.0883) -> (17.86, 88.1645) projected
  circle A145 centre (7.891, 75.5745) radius 2.55
  circle A146 centre (26.591, 75.5745) radius 2.55
  circle A147 centre (45.291, 75.5745) radius 2.55
  line L172 (15.59, 80.0195) -> (52.99, 80.0195) construction
  arc A148 (31.3611, 79.3703) -> (35.4766, 77.2641) centre (34.29, 80.0195) ccw construction
  line L173 (34.29, 80.0195) -> (26.591, 75.5745) construction
  line L174 (15.59, 80.0195) -> (7.891, 75.5745) construction
  line L175 (52.99, 80.0195) -> (45.291, 75.5745) construction
  spline S0 degree 2 poles (13.6473, 100.3429) (13.2966, 100.3429) (12.768, 100.4787) (12.5408, 100.5775) knots 0 0 0 1 2 2 2
  line L176 (12.5408, 100.5775) -> (12.5408, 101.3037)
  line L177 (12.5408, 101.3037) -> (12.6099, 101.3037)
  spline S1 degree 2 poles (12.6099, 101.3037) (12.8396, 101.1086) (13.3905, 100.8986) (13.6498, 100.8986) knots 0 0 0 1 2 2 2
  spline S2 degree 2 poles (13.6498, 100.8986) (13.7165, 100.8986) (13.9314, 100.9283) (13.9956, 100.9579) knots 0 0 0 1 2 2 2
  spline S3 degree 2 poles (13.9956, 100.9579) (14.0746, 100.9925) (14.1858, 101.1185) (14.1858, 101.2197) knots 0 0 0 1 2 2 2
  spline S4 degree 2 poles (14.1858, 101.2197) (14.1858, 101.3358) (14.0055, 101.4791) (13.882, 101.5112) knots 0 0 0 1 2 2 2
  spline S5 degree 2 poles (13.882, 101.5112) (13.7264, 101.5532) (13.3732, 101.6248) (13.2175, 101.6792) knots 0 0 0 1 2 2 2
  spline S6 degree 2 poles (13.2175, 101.6792) (12.8643, 101.8027) (12.5581, 102.225) (12.5581, 102.5412) knots 0 0 0 1 2 2 2
  spline S7 degree 2 poles (12.5581, 102.5412) (12.5581, 102.9685) (13.2818, 103.4996) (13.8252, 103.4996) knots 0 0 0 1 2 2 2
  spline S8 degree 2 poles (13.8252, 103.4996) (14.0969, 103.4996) (14.6353, 103.3884) (14.8478, 103.2946) knots 0 0 0 1 2 2 2
  line L178 (14.8478, 103.2946) -> (14.8478, 102.598)
  line L179 (14.8478, 102.598) -> (14.7811, 102.598)
  spline S9 degree 2 poles (14.7811, 102.598) (14.6106, 102.7437) (14.1216, 102.9438) (13.8647, 102.9438) knots 0 0 0 1 2 2 2
  spline S10 degree 2 poles (13.8647, 102.9438) (13.7634, 102.9438) (13.6053, 102.9142) (13.5164, 102.8747) knots 0 0 0 1 2 2 2
  spline S11 degree 2 poles (13.5164, 102.8747) (13.4448, 102.8425) (13.3411, 102.7141) (13.3411, 102.6351) knots 0 0 0 1 2 2 2
  spline S12 degree 2 poles (13.3411, 102.6351) (13.3411, 102.5165) (13.5065, 102.3806) (13.7437, 102.3263) knots 0 0 0 1 2 2 2
  spline S13 degree 2 poles (13.7437, 102.3263) (13.8968, 102.2917) (14.1809, 102.225) (14.3439, 102.1682) knots 0 0 0 1 2 2 2
  spline S14 degree 2 poles (14.3439, 102.1682) (14.66, 102.0521) (14.9688, 101.6668) (14.9688, 101.3507) knots 0 0 0 1 2 2 2
  spline S15 degree 2 poles (14.9688, 101.3507) (14.9688, 100.8962) (14.255, 100.3429) (13.6473, 100.3429) knots 0 0 0 1 2 2 2
  line L180 (18.4737, 100.3972) -> (17.713, 100.3972)
  line L181 (17.713, 100.3972) -> (17.713, 102.4177)
  line L182 (17.713, 102.4177) -> (17.1597, 101.1135)
  line L183 (17.1597, 101.1135) -> (16.6361, 101.1135)
  line L184 (16.6361, 101.1135) -> (16.0828, 102.4177)
  line L185 (16.0828, 102.4177) -> (16.0828, 100.3972)
  line L186 (16.0828, 100.3972) -> (15.3615, 100.3972)
  line L187 (15.3615, 100.3972) -> (15.3615, 103.4452)
  line L188 (15.3615, 103.4452) -> (16.2433, 103.4452)
  line L189 (16.2433, 103.4452) -> (16.9201, 101.941)
  line L190 (16.9201, 101.941) -> (17.5919, 103.4452)
  line L191 (17.5919, 103.4452) -> (18.4737, 103.4452)
  line L192 (18.4737, 103.4452) -> (18.4737, 100.3972)
  line L193 (34.2591, 100.3429) -> (33.4984, 100.3429)
  line L194 (33.4984, 100.3429) -> (33.4984, 102.3634)
  line L195 (33.4984, 102.3634) -> (32.9451, 101.0592)
  line L196 (32.9451, 101.0592) -> (32.4214, 101.0592)
  line L197 (32.4214, 101.0592) -> (31.8681, 102.3634)
  line L198 (31.8681, 102.3634) -> (31.8681, 100.3429)
  line L199 (31.8681, 100.3429) -> (31.1469, 100.3429)
  line L200 (31.1469, 100.3429) -> (31.1469, 103.3909)
  line L201 (31.1469, 103.3909) -> (32.0287, 103.3909)
  line L202 (32.0287, 103.3909) -> (32.7055, 101.8866)
  line L203 (32.7055, 101.8866) -> (33.3773, 103.3909)
  line L204 (33.3773, 103.3909) -> (34.2591, 103.3909)
  line L205 (34.2591, 103.3909) -> (34.2591, 100.3429)
  spline S16 degree 2 poles (37.6109, 101.8644) (37.6109, 101.4371) (37.238, 100.7653) (36.9539, 100.5849) knots 0 0 0 1 2 2 2
  spline S17 degree 2 poles (36.9539, 100.5849) (36.7168, 100.4318) (36.1586, 100.3429) (35.8449, 100.3429) knots 0 0 0 1 2 2 2
  line L206 (35.8449, 100.3429) -> (34.8914, 100.3429)
  line L207 (34.8914, 100.3429) -> (34.8914, 103.3909)
  line L208 (34.8914, 103.3909) -> (35.835, 103.3909)
  spline S18 degree 2 poles (35.835, 103.3909) (36.1561, 103.3909) (36.7168, 103.3094) (36.9638, 103.1513) knots 0 0 0 1 2 2 2
  spline S19 degree 2 poles (36.9638, 103.1513) (37.2627, 102.9586) (37.6109, 102.3065) (37.6109, 101.8644) knots 0 0 0 1 2 2 2
  spline S20 degree 2 poles (36.8255, 101.8694) (36.8255, 102.1707) (36.618, 102.6005) (36.4056, 102.7215) knots 0 0 0 1 2 2 2
  spline S21 degree 2 poles (36.4056, 102.7215) (36.25, 102.8055) (35.9091, 102.8228) (35.672, 102.8228) knots 0 0 0 1 2 2 2
  line L209 (35.672, 102.8228) -> (35.6572, 102.8228)
  line L210 (35.6572, 102.8228) -> (35.6572, 100.9135)
  line L211 (35.6572, 100.9135) -> (35.672, 100.9135)
  spline S22 degree 2 poles (35.672, 100.9135) (35.9289, 100.9135) (36.2821, 100.9307) (36.4426, 101.032) knots 0 0 0 1 2 2 2
  spline S23 degree 2 poles (36.4426, 101.032) (36.6303, 101.1506) (36.8255, 101.568) (36.8255, 101.8694) knots 0 0 0 1 2 2 2
  line L212 (52.5787, 100.4022) -> (50.5459, 100.4022)
  line L213 (50.5459, 100.4022) -> (50.5459, 103.4502)
  line L214 (50.5459, 103.4502) -> (51.3116, 103.4502)
  line L215 (51.3116, 103.4502) -> (51.3116, 100.9826)
  line L216 (51.3116, 100.9826) -> (52.5787, 100.9826)
  line L217 (52.5787, 100.9826) -> (52.5787, 100.4022)
  spline S24 degree 2 poles (55.4884, 100.5751) (55.2884, 100.4936) (54.6486, 100.3379) (54.3374, 100.3379) knots 0 0 0 1 2 2 2
  spline S25 degree 2 poles (54.3374, 100.3379) (53.6186, 100.3379) (52.7665, 101.1679) (52.7665, 101.9286) knots 0 0 0 1 2 2 2
  spline S26 degree 2 poles (52.7665, 101.9286) (52.7665, 102.6449) (53.6186, 103.5094) (54.3596, 103.5094) knots 0 0 0 1 2 2 2
  spline S27 degree 2 poles (54.3596, 103.5094) (54.7425, 103.5094) (55.2217, 103.3637) (55.4761, 103.2402) knots 0 0 0 1 2 2 2
  line L218 (55.4761, 103.2402) -> (55.4761, 102.5239)
  line L219 (55.4761, 102.5239) -> (55.4069, 102.5239)
  spline S28 degree 2 poles (55.4069, 102.5239) (55.3526, 102.5659) (55.1451, 102.7265) (55.0463, 102.7808) knots 0 0 0 1 2 2 2
  spline S29 degree 2 poles (55.0463, 102.7808) (54.9327, 102.8475) (54.6313, 102.9413) (54.4634, 102.9413) knots 0 0 0 1 2 2 2
  spline S30 degree 2 poles (54.4634, 102.9413) (54.2682, 102.9413) (53.9447, 102.8178) (53.8187, 102.6919) knots 0 0 0 1 2 2 2
  spline S31 degree 2 poles (53.8187, 102.6919) (53.6977, 102.5684) (53.5569, 102.1905) (53.5569, 101.941) knots 0 0 0 1 2 2 2
  spline S32 degree 2 poles (53.5569, 101.941) (53.5569, 101.4075) (54.0929, 100.8986) (54.5548, 100.8986) knots 0 0 0 1 2 2 2
  spline S33 degree 2 poles (54.5548, 100.8986) (54.5967, 100.8986) (54.7054, 100.9036) (54.7474, 100.906) knots 0 0 0 1 2 2 2
  line L220 (54.7474, 100.906) -> (54.7474, 101.5063)
  line L221 (54.7474, 101.5063) -> (54.1571, 101.5063)
  line L222 (54.1571, 101.5063) -> (54.1571, 102.0768)
  line L223 (54.1571, 102.0768) -> (55.4884, 102.0768)
  line L224 (55.4884, 102.0768) -> (55.4884, 100.5751)
  line L225 (17.0251, 68.4965) -> (16.1408, 68.4965)
  line L226 (16.1408, 68.4965) -> (15.5529, 69.4672)
  line L227 (15.5529, 69.4672) -> (14.9527, 68.4965)
  line L228 (14.9527, 68.4965) -> (14.1055, 68.4965)
  line L229 (14.1055, 68.4965) -> (15.096, 70.0304)
  line L230 (15.096, 70.0304) -> (14.145, 71.5445)
  line L231 (14.145, 71.5445) -> (15.0293, 71.5445)
  line L232 (15.0293, 71.5445) -> (15.5801, 70.6232)
  line L233 (15.5801, 70.6232) -> (16.1458, 71.5445)
  line L234 (16.1458, 71.5445) -> (16.993, 71.5445)
  line L235 (16.993, 71.5445) -> (16.0371, 70.0625)
  line L236 (16.0371, 70.0625) -> (17.0251, 68.4965)
  line L237 (35.6967, 71.5445) -> (34.6444, 69.7685)
  line L238 (34.6444, 69.7685) -> (34.6444, 68.4965)
  line L239 (34.6444, 68.4965) -> (33.8787, 68.4965)
  line L240 (33.8787, 68.4965) -> (33.8787, 69.7315)
  line L241 (33.8787, 69.7315) -> (32.8092, 71.5445)
  line L242 (32.8092, 71.5445) -> (33.6811, 71.5445)
  line L243 (33.6811, 71.5445) -> (34.2764, 70.4577)
  line L244 (34.2764, 70.4577) -> (34.8519, 71.5445)
  line L245 (34.8519, 71.5445) -> (35.6967, 71.5445)
  line L246 (51.7673, 71.5445) -> (54.183, 71.5445)
  line L247 (54.183, 71.5445) -> (54.183, 70.9739)
  line L248 (54.183, 70.9739) -> (52.7776, 69.0769)
  line L249 (52.7776, 69.0769) -> (54.1089, 69.0769)
  line L250 (54.1089, 69.0769) -> (54.1089, 68.4965)
  line L251 (54.1089, 68.4965) -> (51.8489, 68.4965)
  line L252 (51.8489, 68.4965) -> (51.8489, 69.0769)
  line L253 (51.8489, 69.0769) -> (53.2494, 70.964)
  line L254 (53.2494, 70.964) -> (51.7673, 70.964)
  line L255 (51.7673, 70.964) -> (51.7673, 71.5445)
  point P0 (52.99, 100.3429)
  point P1 (34.29, 100.3429)
  point P2 (15.59, 100.3429)
  point P3 (34.29, 71.5445)
  point P4 (52.99, 71.5445)
  point P5 (15.59, 71.5445)
  dimension "d0" = 68.58
  dimension "d1" = 107.95
  dimension "d63" = 5.1
  dimension "d64" = 30
  dimension "d65" = 30
  dimension "d66" = 30
  dimension "d67" = 8.89
  dimension "d70" = 1
  dimension "d71" = 1
  constraints: 8 end point, 7 midpoint, 6 vertical alignment, 4 collinear, 3 centre point, 2 equal radius, 2 parallel, 1 horizontal, 12 other
  measures "d63" diameter of A145
  measures "d64" angle of L172 L175
  measures "d65" angle of L172 L173
  measures "d66" angle of L172 L174
  measures "d67" distance of L173.start L173.end
  measures "d70" distance between parallel lines of L52 L4
  measures "d71" distance from line of L121.end L18
extrude "Extrusion8" cut sketch "Sketch7" against normal through all contours A145 | A146 | A147
extrude "Extrusion9" cut sketch "Sketch7" against normal blind 0.5 contours S0 L176 L177 S1 S2 S3 S4 S5 S6 S7 S8 L178 L179 S9 S10 S11 S12 S13 S14 S15 | L180 L181 L182 L183 L184 L185 L186 L187 L188 L189 L190 L191 L192 | L193 L194 L195 L196 L197 L198 L199 L200 L201 L202 L203 L204 L205 | S16 S17 L206 L207 L208 S18 S19 | L212 L213 L214 L215 L216 L217 | S24 S25 S26 S27 L218 L219 S28 S29 S30 S31 S32 S33 L220 L221 L222 L223 L224 | L225 L226 L227 L228 L229 L230 L231 L232 L233 L234 L235 L236 | L237 L238 L239 L240 L241 L242 L243 L244 L245 | L246 L247 L248 L249 L250 L251 L252 L253 L254 L255